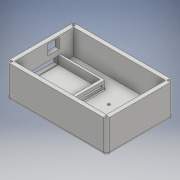
# Autodesk Inventor part: Back Plate test04
Saved by Autodesk Inventor 2018 (Build 220112000, 112)
## iProperties
Created: 2022-01-10
Part Number: Back Plate test04
Material: Generic
Document SubType Name: Modeling
Designer: Stewart Alexander
Density: 1 g/cm^3
Appearance: Default
Author: Stewart Alexander
Autodesk Inventor part; units mm, degrees
ref_plane "YZ Plane" through (0, 0, 0) normal (1, 0, 0) x (0, 1, 0)
ref_plane "XZ Plane" through (0, 0, 0) normal (0, 1, 0) x (-1, 0, 0)
ref_plane "XY Plane" through (0, 0, 0) normal (0, 0, 1) x (1, 0, 0)
sketch "Arduino Uno" plane through (0, 0, 0) normal (0, 0, 1) x (1, 0, 0)
  line L0 (0, 0) -> (68.6, 0)
  line L1 (68.6, 0) -> (68.6, 53.3)
  line L2 (68.6, 53.3) -> (0, 53.3)
  line L3 (0, 53.3) -> (0, 0)
  circle A0 centre (14, 2.5) radius 1.6
  circle A1 centre (15.3, 50.7) radius 1.6
  circle A2 centre (66.1, 5.1) radius 1.6
  circle A3 centre (66.1, 33) radius 1.6
  dimension "d6" = 68.6
  dimension "d7" = 53.3
  dimension "d8" = 3.2
  dimension "d12" = 14
  dimension "d13" = 2.5
  dimension "d14" = 3.2
  dimension "d15" = 1.3
  dimension "d16" = 3.2
  dimension "d18" = 2.5
  dimension "d19" = 5.1
  dimension "d20" = 3.2
  dimension "d21" = 27.9
  dimension "d22" = 2.5
  dimension "d26" = 2.6
  constraints: 8 end point, 4 centre point, 2 parallel, 1 horizontal, 1 perpendicular
  measures "d6" distance of L2.end L1.end
  measures "d7" distance of L0.end L1.end
  measures "d8" diameter of A0
  measures "d12" distance from line of L3 A0.centre
  measures "d13" distance from line of L0 A0.centre
  measures "d14" diameter of A1
  measures "d15" horizontal distance of A0.centre A1.centre
  measures "d16" diameter of A2
  measures "d18" distance from line of L1 A2.centre
  measures "d19" distance from line of L0 A2.centre
  measures "d20" diameter of A3
  measures "d21" distance of A2.centre A3.centre
  measures "d22" distance from line of L1 A3.centre
  measures "d26" distance from line of L2 A1.centre
sketch "Sketch2" plane through (0, 0, 0) normal (0, 0, 1) x (1, 0, 0)
  line L0 (-7.6136, -10.2044) -> (-7.6136, 63.0956)
  line L1 (-7.6136, 63.0956) -> (106.3864, 63.0956)
  line L2 (106.3864, 63.0956) -> (106.3864, -10.2044)
  line L3 (106.3864, -10.2044) -> (-7.6136, -10.2044)
  dimension "d29" = 114
  dimension "d39" = 73.3
  constraints: 8 end point, 3 perpendicular
  measures "d29" distance of L0.end L1.end
  measures "d39" distance of L0.start L0.end
extrude "Back Plate" add sketch "Sketch2" against normal blind 10
extrude "Uno Mounting Holes" cut sketch "Arduino Uno" against normal blind 5 contours A0 | A1 | A2 | A3
sketch "3.5\" TFT LCD Screen" plane through (0, 0, 0) normal (0, 0, 1) x (1, 0, 0)
  line L0 (88.6005, 0.0003) -> (88.6005, 53.3003)
  line L1 (88.6005, 53.3003) -> (10.6005, 53.3003)
  line L2 (10.6005, 53.3003) -> (10.6005, 0.0003)
  line L3 (10.6005, 0.0003) -> (88.6005, 0.0003)
  circle A0 centre (66.1, 5.1) radius 1.6 projected
  circle A1 centre (14, 2.5) radius 1.6 projected
  circle A2 centre (15.3, 50.7) radius 1.6 projected
  circle A3 centre (66.1, 33) radius 1.6 projected
  line L4 (-7.6136, -10.2044) -> (-7.6136, 63.0956) projected
  line L5 (106.3864, -10.2044) -> (-7.6136, -10.2044) projected
  line L6 (106.3864, 63.0956) -> (106.3864, -10.2044) projected
  line L7 (-7.6136, 63.0956) -> (106.3864, 63.0956) projected
  point P0 (0, 0)
  point P1 (68.6, 0)
  dimension "d35" = 78
  dimension "d36" = 53.3
  dimension "d37" = 78
  dimension "d38" = 53.3
  constraints: 8 end point
  measures "d35" distance of L2.end L0.start
  measures "d36" distance of L1.end L2.end
  measures "d37" distance of L0.end L1.end
  measures "d38" distance of L0.start L0.end
sketch "SD Card Slot" plane through (0, 0, 0) normal (0, 0, 1) x (1, 0, 0)
  line L0 (43.3864, 9.1) -> (-7.6136, 9.1)
  line L1 (-7.6136, 9.1) -> (-7.6136, 44.1)
  line L2 (-7.6136, 44.1) -> (43.3864, 44.1)
  line L3 (43.3864, 44.1) -> (43.3864, 9.1)
  circle A0 centre (14, 2.5) radius 1.6 projected
  line L4 (-7.6136, -10.2044) -> (-7.6136, 63.0956) projected
  circle A1 centre (15.3, 50.7) radius 1.6 projected
  point P0 (0, 0)
  dimension "d41" = 35
  dimension "d42" = 51
  dimension "d44" = 6.6
  dimension "d45" = 0
  constraints: 8 end point, 2 parallel, 1 horizontal, 1 perpendicular
  measures "d41" distance of L0.end L1.end
  measures "d42" distance of L0.start L0.end
  measures "d44" distance from line of L0 A0.centre
  measures "d45" distance between parallel lines of L4 L1
sketch "Sketch5" plane through (0, 0, 0) normal (0, 0, 1) x (1, 0, 0)
  line L0 (43.3864, 9.1) -> (-7.6136, 9.1) projected
  line L1 (43.3864, 44.1) -> (43.3864, 9.1) projected
  line L2 (-7.6136, 44.1) -> (43.3864, 44.1) projected
  line L3 (-7.6136, 9.1) -> (-7.6136, 44.1) projected
  line L4 (43.8864, 8.6) -> (43.8864, 44.6)
  line L5 (43.8864, 8.6) -> (-7.6136, 8.6)
  line L6 (-7.6136, -10.2044) -> (-7.6136, 63.0956) projected
  line L7 (43.8864, 44.6) -> (-7.6136, 44.6)
  line L8 (-7.6136, 44.6) -> (-7.6136, 47.1)
  line L9 (-7.6136, 47.1) -> (47.3864, 47.1)
  line L10 (-7.6136, 8.6) -> (-7.6136, 6.1)
  line L11 (-7.6136, 6.1) -> (47.3864, 6.1)
  line L12 (47.3864, 6.1) -> (47.3864, 47.1)
  point P0 (0, 0)
  dimension "d47" = 2.5
  dimension "d48" = 55
  dimension "d49" = 2.5
  dimension "d72" = 0.5
  dimension "d73" = 0.5
  dimension "d74" = 0.5
  constraints: 16 end point, 4 perpendicular, 3 point on line, 1 horizontal, 1 parallel
  measures "d47" distance of L7.end L8.end
  measures "d48" distance of L8.end L9.end
  measures "d49" distance of L5.end L10.end
  measures "d72" distance between parallel lines of L1 L4
  measures "d73" distance between parallel lines of L0 L5
  measures "d74" distance between parallel lines of L2 L7
extrude "SD Card Slot Slot" add sketch "Sketch5" along normal blind 10 contours L5 L4 L7 L6 L9 L12 L11
sketch "Sketch6" plane through (47.3864, 6.1, 0) normal (1, 0, 0) x (0, 0, -1)
  line L0 (0, 41) -> (0, 0) projected
  line L1 (0, 41) -> (-10, 41) projected
  line L2 (-10, 0) -> (-10, 41) projected
  line L3 (0, 0) -> (-10, 0) projected
  line L4 (-6, 37) -> (-4, 37)
  line L5 (-4, 37) -> (-4, 4)
  line L6 (-4, 4) -> (-6, 4)
  line L7 (-6, 4) -> (-6, 37)
  point P0 (0, -6.1)
  dimension "d52" = 4
  constraints: 8 end point, 3 other
  measures "d52" distance between parallel lines of L2 L7
extrude "SD Ribbon Slot" cut sketch "Sketch6" against normal through all contours L4 L5 L6 L7
fillet "1.2mm Fillet" radius 1.2 7 edges at (19.8864, 47.1, 0) (19.8864, 6.1, 0) (47.3864, 26.6, 0) (47.3864, 6.1, 5) (47.3864, 47.1, 5) (43.8864, 44.6, 5) (43.8864, 8.6, 5)
sketch "Sketch7" plane through (0, 0, 0) normal (0, 0, 1) x (1, 0, 0)
  line L0 (106.3864, -10.2044) -> (101.3864, -10.2044)
  line L1 (101.3864, -10.2044) -> (101.3864, -5.2044)
  line L2 (101.3864, -5.2044) -> (106.3864, -5.2044)
  line L3 (106.3864, -5.2044) -> (106.3864, -10.2044)
  line L4 (49.3864, -10.2044) -> (49.3864, 80.0118)
  line L5 (-7.6136, 63.0956) -> (106.3864, 63.0956) projected
  line L6 (106.3864, 26.4456) -> (-34.6963, 26.4456)
  line L7 (-7.6136, -10.2044) -> (-2.6136, -10.2044)
  line L8 (-2.6136, -10.2044) -> (-2.6136, -5.2044)
  line L9 (-2.6136, -5.2044) -> (-7.6136, -5.2044)
  line L10 (-7.6136, -5.2044) -> (-7.6136, -10.2044)
  line L11 (106.3864, 63.0956) -> (101.3864, 63.0956)
  line L12 (101.3864, 63.0956) -> (101.3864, 58.0956)
  line L13 (101.3864, 58.0956) -> (106.3864, 58.0956)
  line L14 (106.3864, 58.0956) -> (106.3864, 63.0956)
  line L15 (-7.6136, 63.0956) -> (-2.6136, 63.0956)
  line L16 (-2.6136, 63.0956) -> (-2.6136, 58.0956)
  line L17 (-2.6136, 58.0956) -> (-7.6136, 58.0956)
  line L18 (-7.6136, 58.0956) -> (-7.6136, 63.0956)
  point P0 (0, 0)
  point P1 (0, 52.8913)
  dimension "d56" = 5
  dimension "d57" = 5
  dimension "d58" = 57
  dimension "d59" = 36.65
  constraints: 36 end point, 11 symmetric about line, 2 parallel, 2 perpendicular, 1 horizontal
  measures "d56" distance of L1.end L2.end
  measures "d57" distance of L0.end L1.end
  measures "d58" distance of L0.start L4.start
  measures "d59" distance of L0.start L6.start
extrude "Pillars" [suppressed]
sketch "Sketch8" plane through (0, 0, 31) normal (0, 0, 1) x (1, 0, 0)
  line L0 (101.3864, -10.2044) -> (-2.6136, -10.2044) projected
  line L1 (-7.6136, -5.2044) -> (-2.6136, -5.2044) projected
  line L2 (101.3864, -10.2044) -> (-2.6136, -10.2044)
  line L3 (-2.6136, -10.2044) -> (-2.6136, -5.2044)
  line L4 (-2.6136, -5.2044) -> (101.3864, -5.2044)
  line L5 (101.3864, -5.2044) -> (101.3864, -10.2044)
  line L6 (101.3864, 63.0956) -> (101.3864, 58.0956) projected
  line L7 (106.3864, 63.0956) -> (106.3864, -10.2044) projected
  line L8 (101.3864, 58.0956) -> (106.3864, 58.0956)
  line L9 (106.3864, 58.0956) -> (106.3864, -5.2044)
  line L10 (106.3864, -5.2044) -> (101.3864, -5.2044)
  line L11 (101.3864, -5.2044) -> (101.3864, 58.0956)
  line L12 (-7.6136, 58.0956) -> (-2.6136, 58.0956) projected
  line L13 (-7.6136, 63.0956) -> (106.3864, 63.0956) projected
  line L14 (-2.6136, 58.0956) -> (101.3864, 58.0956)
  line L15 (101.3864, 58.0956) -> (101.3864, 63.0956)
  line L16 (101.3864, 63.0956) -> (-2.6136, 63.0956)
  line L17 (-2.6136, 63.0956) -> (-2.6136, 58.0956)
  line L18 (-2.6136, 58.0956) -> (-7.6136, 58.0956)
  line L19 (-7.6136, 58.0956) -> (-7.6136, -5.2044)
  line L20 (-7.6136, -5.2044) -> (-2.6136, -5.2044)
  line L21 (-2.6136, -5.2044) -> (-2.6136, 58.0956)
  point P0 (0, 0)
  constraints: 32 end point, 8 parallel, 4 horizontal, 4 perpendicular, 3 point on line
extrude "Beams (Will they print?)" [suppressed]
sketch "Sketch9" plane through (0, 0, 0) normal (0, 0, 1) x (1, 0, 0)
  line L0 (106.3864, 63.0956) -> (106.3864, -10.2044) projected
  line L1 (-7.6136, -10.2044) -> (-7.6136, 63.0956) projected
  line L2 (106.3864, -10.2044) -> (-7.6136, -10.2044)
  line L3 (-7.6136, -10.2044) -> (-7.6136, 63.0956)
  line L4 (-7.6136, 63.0956) -> (106.3864, 63.0956) projected
  line L5 (-7.6136, 63.0956) -> (106.3864, 63.0956)
  line L6 (106.3864, 63.0956) -> (106.3864, -10.2044)
  line L7 (106.3864, -10.2044) -> (106.3864, -15.2044)
  line L8 (106.3864, -15.2044) -> (-7.6136, -15.2044)
  line L9 (-7.6136, -15.2044) -> (-12.6136, -15.2044)
  line L10 (-12.6136, -15.2044) -> (-12.6136, 63.0956)
  line L11 (-12.6136, 63.0956) -> (-12.6136, 68.0956)
  line L12 (-12.6136, 68.0956) -> (106.3864, 68.0956)
  line L13 (106.3864, 68.0956) -> (111.3864, 68.0956)
  line L14 (111.3864, 68.0956) -> (111.3864, -15.2044)
  line L15 (111.3864, -15.2044) -> (106.3864, -15.2044)
  point P0 (0, 0)
  dimension "d64" = 5
  dimension "d65" = 5
  dimension "d66" = 5
  dimension "d67" = 5
  constraints: 26 end point, 8 point on line, 6 perpendicular, 2 collinear, 1 horizontal
  measures "d64" distance of L0.end L7.end
  measures "d65" distance of L8.end L9.end
  measures "d66" distance of L10.end L11.end
  measures "d67" distance of L12.end L13.end
extrude "Outer Walls (5mm Offset)" add sketch "Sketch9" along normal blind 31 and the other way blind 10
extrude "Extrusion9" [suppressed]
sketch "Sketch10" plane through (-12.6136, -15.2044, 31) normal (-1, 0, 0) x (0, 0, 1)
  line L0 (-31, 58.6044) -> (-21, 58.6044) projected
  line L1 (-29.8, 61.1044) -> (-29.8, 22.5044) projected
  line L2 (-21, 58.6044) -> (-21, 25.0044) projected
  line L3 (-21, 58.6044) -> (-21, 25.0044)
  line L4 (-21, 25.0044) -> (-29.8, 25.0044)
  line L5 (-29.8, 25.0044) -> (-29.8, 58.6044)
  line L6 (-29.8, 58.6044) -> (-21, 58.6044)
  line L7 (-31, 63.5044) -> (-31, 78.3) projected
  line L8 (-13.6, 59.5047) -> (-2.9, 59.5047)
  line L9 (-2.9, 59.5047) -> (-2.9, 47.5047)
  line L10 (-2.9, 47.5047) -> (-13.6, 47.5047)
  line L11 (-13.6, 47.5047) -> (-13.6, 59.5047)
  line L12 (-1.9, 46.5047) -> (-1.9, 60.5047)
  line L13 (-1.9, 60.5047) -> (-14.6, 60.5047)
  line L14 (-14.6, 60.5047) -> (-14.6, 46.5047)
  line L15 (-14.6, 46.5047) -> (-1.9, 46.5047)
  point P0 (-31, 15.2044)
  point P1 (-31, 68.5047)
  dimension "d82" = 10.7
  dimension "d83" = 12
  dimension "d84" = 1
  constraints: 24 end point, 7 perpendicular, 3 point on line, 2 collinear, 1 horizontal, 3 other
  measures "d82" distance of L8.start L8.end
  measures "d83" distance of L8.end L9.end
  measures "d84" distance between parallel lines of L9 L12
extrude "SD Card Opening" cut sketch "Sketch10" against normal blind 5 contours L0 L2 L4 L1 | L8 L9 L10 L11 | L15 L14 L13 L12
fillet "4mm Fillet" radius 4 8 edges at (-12.6136, 68.0956, 10.5) (-12.6136, -15.2044, 10.5) (111.3864, -15.2044, 10.5) (111.3864, 68.0956, 10.5) (49.3864, 68.0956, -10) (-12.6136, 26.4456, -10) (49.3864, -15.2044, -10) (111.3864, 26.4456, -10)
sketch "Sketch11" plane through (0, 0, 0) normal (0, 0, 1) x (1, 0, 0)
  line L0 (98.4778, 47.4456) -> (98.4778, 5.4456) construction
  line L1 (98.4778, 5.4456) -> (86.054, 5.4456) construction
  line L2 (86.054, 5.4456) -> (86.054, 47.4456) construction
  line L3 (86.054, 47.4456) -> (98.4778, 47.4456) construction
  line L4 (-8.6136, 68.0956) -> (107.3864, 68.0956) projected
  line L5 (107.3864, 68.0956) -> (107.3864, 26.4456)
  line L6 (107.3864, 26.4456) -> (48.9636, 26.4456)
  line L7 (94.9648, 45.4666) -> (98.011, 44.7345)
  line L8 (98.011, 44.7345) -> (98.011, 45.124)
  line L9 (98.011, 45.124) -> (98.4778, 45.0166)
  line L10 (98.4778, 45.0166) -> (98.4778, 42.1518)
  line L11 (98.4778, 42.1518) -> (97.2789, 42.454)
  line L12 (97.2789, 42.454) -> (97.2789, 42.9276)
  line L13 (97.2789, 42.9276) -> (98.011, 42.7429)
  line L14 (98.011, 42.7429) -> (98.011, 44.1534)
  line L15 (98.011, 44.1534) -> (96.7952, 44.4456)
  line L16 (96.7952, 44.4456) -> (96.7952, 43.25)
  line L17 (96.7952, 43.25) -> (96.3284, 43.3575)
  line L18 (96.3284, 43.3575) -> (96.3284, 44.5565)
  line L19 (96.3284, 44.5565) -> (94.9648, 44.8856)
  line L20 (94.9648, 44.8856) -> (94.9648, 44.4591)
  line L21 (94.9648, 44.4591) -> (94.498, 44.5665)
  line L22 (94.498, 44.5665) -> (94.498, 45.9301)
  line L23 (94.498, 45.9301) -> (94.9648, 45.8226)
  line L24 (94.9648, 45.8226) -> (94.9648, 45.4666)
  spline S0 degree 2 poles (95.613, 42.5313) (96.0396, 42.5313) (96.8255, 42.1316) (97.3427, 41.3323) (97.3427, 40.8352) knots 0 0 0 1 2 3 3 3
  spline S1 degree 2 poles (97.3427, 40.8352) (97.3427, 40.2575) (96.6676, 39.6362) (96.1538, 39.6362) knots 0 0 0 1 2 2 2
  spline S2 degree 2 poles (96.1538, 39.6362) (95.7474, 39.6362) (94.8943, 40.0325) (94.4174, 40.8554) (94.4174, 41.3155) knots 0 0 0 1 2 3 3 3
  spline S3 degree 2 poles (94.4174, 41.3155) (94.4174, 41.8495) (95.0488, 42.5313) (95.613, 42.5313) knots 0 0 0 1 2 2 2
  spline S4 degree 2 poles (95.6634, 41.9536) (94.9145, 41.9536) (94.9145, 41.2617) knots 0 0 0 1 1 1
  spline S5 degree 2 poles (94.9145, 41.2617) (94.9145, 40.7748) (95.66, 40.187) (96.1504, 40.187) knots 0 0 0 1 2 2 2
  spline S6 degree 2 poles (96.1504, 40.187) (96.4661, 40.187) (96.8456, 40.59) (96.8456, 40.9192) knots 0 0 0 1 2 2 2
  spline S7 degree 2 poles (96.8456, 40.9192) (96.8456, 41.3894) (96.1235, 41.9536) (95.6634, 41.9536) knots 0 0 0 1 2 2 2
  line L25 (94.9648, 38.5581) -> (94.9648, 38.1014)
  line L26 (94.9648, 38.1014) -> (94.498, 38.2122)
  line L27 (94.498, 38.2122) -> (94.498, 39.5489)
  line L28 (94.498, 39.5489) -> (94.9648, 39.4414)
  line L29 (94.9648, 39.4414) -> (94.9648, 39.0787)
  line L30 (94.9648, 39.0787) -> (96.7986, 38.6656)
  line L31 (96.7986, 38.6656) -> (96.7986, 39.0955)
  line L32 (96.7986, 39.0955) -> (97.2654, 38.9813)
  line L33 (97.2654, 38.9813) -> (97.2654, 38.0846)
  line L34 (97.2654, 38.0846) -> (96.4829, 38.2626)
  spline S8 degree 2 poles (96.4829, 38.2626) (96.9161, 38.0006) (97.3091, 37.4028) (97.3091, 36.9998) knots 0 0 0 1 2 2 2
  line L35 (97.3091, 36.9998) -> (97.3091, 36.8755)
  line L36 (97.3091, 36.8755) -> (96.7986, 36.9964)
  spline S9 degree 2 poles (96.7986, 36.9964) (96.8087, 37.0737) (96.8087, 37.1274) knots 0 0 0 1 1 1
  spline S10 degree 2 poles (96.8087, 37.1274) (96.8087, 37.4935) (96.4728, 38.0275) (95.9019, 38.3465) (95.4619, 38.4473) knots 0 0 0 1 2 3 3 3
  line L37 (95.4619, 38.4473) -> (94.9648, 38.5581)
  line L38 (94.9648, 33.2315) -> (94.9648, 32.8856)
  line L39 (94.9648, 32.8856) -> (94.498, 32.983)
  line L40 (94.498, 32.983) -> (94.498, 33.8293)
  line L41 (94.498, 33.8293) -> (94.8842, 33.742)
  spline S11 degree 2 poles (94.8842, 33.742) (94.451, 34.1383) (94.451, 34.6354) knots 0 0 0 1 1 1
  spline S12 degree 2 poles (94.451, 34.6354) (94.451, 34.9578) (94.8909, 35.4683) (95.2604, 35.4683) knots 0 0 0 1 2 2 2
  spline S13 degree 2 poles (95.2604, 35.4683) (95.6768, 35.4683) (96.2243, 34.7932) (96.2243, 34.2962) knots 0 0 0 1 2 2 2
  spline S14 degree 2 poles (96.2243, 34.2962) (96.2243, 33.9099) (96.0228, 33.5271) knots 0 0 0 1 1 1
  line L42 (96.0228, 33.5271) -> (96.3284, 33.4532)
  spline S15 degree 2 poles (96.3284, 33.4532) (96.4896, 33.4162) (96.5568, 33.4162) knots 0 0 0 1 1 1
  spline S16 degree 2 poles (96.5568, 33.4162) (96.7381, 33.4162) (96.9296, 33.7017) (96.9296, 33.9099) knots 0 0 0 1 2 2 2
  spline S17 degree 2 poles (96.9296, 33.9099) (96.9296, 34.313) (96.5366, 34.5884) knots 0 0 0 1 1 1
  line L43 (96.5366, 34.5884) -> (96.7348, 35.0216)
  spline S18 degree 2 poles (96.7348, 35.0216) (96.9934, 34.8537) (97.3427, 34.2021) (97.3427, 33.8159) knots 0 0 0 1 2 2 2
  spline S19 degree 2 poles (97.3427, 33.8159) (97.3427, 33.3793) (96.9665, 32.899) (96.6642, 32.899) knots 0 0 0 1 2 2 2
  spline S20 degree 2 poles (96.6642, 32.899) (96.4795, 32.899) (96.1941, 32.9628) knots 0 0 0 1 1 1
  line L44 (96.1941, 32.9628) -> (94.9648, 33.2315)
  line L45 (95.6433, 33.6077) -> (95.7004, 33.7319)
  spline S21 degree 2 poles (95.7004, 33.7319) (95.828, 34.0174) (95.828, 34.2559) knots 0 0 0 1 1 1
  spline S22 degree 2 poles (95.828, 34.2559) (95.828, 34.5716) (95.5022, 34.9544) (95.2772, 34.9544) knots 0 0 0 1 2 2 2
  spline S23 degree 2 poles (95.2772, 34.9544) (95.0857, 34.9544) (94.8641, 34.6891) (94.8641, 34.4708) knots 0 0 0 1 2 2 2
  spline S24 degree 2 poles (94.8641, 34.4708) (94.8641, 34.135) (95.2268, 33.7118) knots 0 0 0 1 1 1
  line L46 (95.2268, 33.7118) -> (95.6433, 33.6077)
  line L47 (94.9648, 32.1635) -> (98.011, 31.4314)
  line L48 (98.011, 31.4314) -> (98.011, 31.8041)
  line L49 (98.011, 31.8041) -> (98.4778, 31.6967)
  line L50 (98.4778, 31.6967) -> (98.4778, 30.7999)
  line L51 (98.4778, 30.7999) -> (94.9648, 31.6463)
  line L52 (94.9648, 31.6463) -> (94.9648, 31.2701)
  line L53 (94.9648, 31.2701) -> (94.498, 31.381)
  line L54 (94.498, 31.381) -> (94.498, 32.59)
  line L55 (94.498, 32.59) -> (94.9648, 32.4826)
  line L56 (94.9648, 32.4826) -> (94.9648, 32.1635)
  line L57 (94.9648, 30.5178) -> (98.011, 29.7857)
  line L58 (98.011, 29.7857) -> (98.011, 30.1585)
  line L59 (98.011, 30.1585) -> (98.4778, 30.051)
  line L60 (98.4778, 30.051) -> (98.4778, 29.1543)
  line L61 (98.4778, 29.1543) -> (94.9648, 30.0006)
  line L62 (94.9648, 30.0006) -> (94.9648, 29.6245)
  line L63 (94.9648, 29.6245) -> (94.498, 29.7353)
  line L64 (94.498, 29.7353) -> (94.498, 30.9444)
  line L65 (94.498, 30.9444) -> (94.9648, 30.8369)
  line L66 (94.9648, 30.8369) -> (94.9648, 30.5178)
  line L67 (97.2654, 26.4204) -> (97.2654, 26.0208)
  line L68 (97.2654, 26.0208) -> (96.7986, 26.1282)
  line L69 (96.7986, 26.1282) -> (96.7986, 26.5313)
  line L70 (96.7986, 26.5313) -> (95.4955, 26.847)
  spline S25 degree 2 poles (95.4955, 26.847) (95.1428, 26.9343) (95.0555, 26.9343) knots 0 0 0 1 1 1
  spline S26 degree 2 poles (95.0555, 26.9343) (94.8607, 26.9343) (94.8607, 26.7261) knots 0 0 0 1 1 1
  spline S27 degree 2 poles (94.8607, 26.7261) (94.8607, 26.585) (95.0219, 26.2962) knots 0 0 0 1 1 1
  line L71 (95.0219, 26.2962) -> (94.545, 26.407)
  spline S28 degree 2 poles (94.545, 26.407) (94.4174, 26.669) (94.4174, 26.9175) knots 0 0 0 1 1 1
  spline S29 degree 2 poles (94.4174, 26.9175) (94.4174, 27.1526) (94.7197, 27.4448) (94.9951, 27.4448) knots 0 0 0 1 2 2 2
  spline S30 degree 2 poles (94.9951, 27.4448) (95.1831, 27.4448) (95.8179, 27.2869) knots 0 0 0 1 1 1
  line L72 (95.8179, 27.2869) -> (96.7986, 27.0518)
  line L73 (96.7986, 27.0518) -> (96.7986, 27.3575)
  line L74 (96.7986, 27.3575) -> (97.2654, 27.25)
  line L75 (97.2654, 27.25) -> (97.2654, 26.9376)
  line L76 (97.2654, 26.9376) -> (97.8162, 26.8033)
  line L77 (97.8162, 26.8033) -> (98.3099, 26.1652)
  line L78 (98.3099, 26.1652) -> (97.2654, 26.4204)
  line L79 (94.9648, 23.5691) -> (94.9648, 23.156)
  line L80 (94.9648, 23.156) -> (94.498, 23.2668)
  line L81 (94.498, 23.2668) -> (94.498, 24.2005)
  line L82 (94.498, 24.2005) -> (96.0328, 23.8377)
  spline S31 degree 2 poles (96.0328, 23.8377) (96.4459, 23.7437) (96.5333, 23.7437) knots 0 0 0 1 1 1
  spline S32 degree 2 poles (96.5333, 23.7437) (96.8187, 23.7437) (96.8187, 24.0392) knots 0 0 0 1 1 1
  spline S33 degree 2 poles (96.8187, 24.0392) (96.8187, 24.3146) (96.4459, 24.8621) knots 0 0 0 1 1 1
  line L83 (96.4459, 24.8621) -> (94.9648, 25.2214)
  line L84 (94.9648, 25.2214) -> (94.9648, 24.8083)
  line L85 (94.9648, 24.8083) -> (94.498, 24.9158)
  line L86 (94.498, 24.9158) -> (94.498, 26.1786)
  line L87 (94.498, 26.1786) -> (94.9648, 26.0712)
  line L88 (94.9648, 26.0712) -> (94.9648, 25.7387)
  line L89 (94.9648, 25.7387) -> (98.011, 25.0065)
  line L90 (98.011, 25.0065) -> (98.011, 25.3726)
  line L91 (98.011, 25.3726) -> (98.4778, 25.2651)
  line L92 (98.4778, 25.2651) -> (98.4778, 24.3751)
  line L93 (98.4778, 24.3751) -> (96.9396, 24.7445)
  spline S34 degree 2 poles (96.9396, 24.7445) (97.3091, 24.224) (97.3091, 23.8478) knots 0 0 0 1 1 1
  spline S35 degree 2 poles (97.3091, 23.8478) (97.3091, 23.5388) (96.9161, 23.213) (96.6676, 23.213) knots 0 0 0 1 2 2 2
  spline S36 degree 2 poles (96.6676, 23.213) (96.4829, 23.213) (95.9858, 23.3306) knots 0 0 0 1 1 1
  line L94 (95.9858, 23.3306) -> (94.9648, 23.5691)
  line L95 (95.7541, 19.8579) -> (95.7541, 22.0308)
  spline S37 degree 2 poles (95.7541, 22.0308) (95.6701, 22.051) (95.5962, 22.051) knots 0 0 0 1 1 1
  spline S38 degree 2 poles (95.5962, 22.051) (95.2537, 22.051) (94.8708, 21.6581) (94.8708, 21.3591) knots 0 0 0 1 2 2 2
  spline S39 degree 2 poles (94.8708, 21.3591) (94.8708, 20.946) (95.2637, 20.6572) knots 0 0 0 1 1 1
  line L96 (95.2637, 20.6572) -> (95.032, 20.1165)
  spline S40 degree 2 poles (95.032, 20.1165) (94.7633, 20.2811) (94.4174, 20.9662) (94.4174, 21.3558) knots 0 0 0 1 2 2 2
  spline S41 degree 2 poles (94.4174, 21.3558) (94.4174, 21.9536) (95.1093, 22.6152) (95.65, 22.6152) knots 0 0 0 1 2 2 2
  spline S42 degree 2 poles (95.65, 22.6152) (96.0832, 22.6152) (96.8523, 22.1786) (97.3427, 21.4465) (97.3427, 21.0099) knots 0 0 0 1 2 3 3 3
  spline S43 degree 2 poles (97.3427, 21.0099) (97.3427, 20.4826) (96.6542, 19.8176) (96.0967, 19.8176) knots 0 0 0 1 2 2 2
  spline S44 degree 2 poles (96.0967, 19.8176) (95.9187, 19.8176) (95.7541, 19.8579) knots 0 0 0 1 1 1
  spline S45 degree 2 poles (96.1437, 20.3482) (96.231, 20.3382) (96.2881, 20.3382) knots 0 0 0 1 1 1
  spline S46 degree 2 poles (96.2881, 20.3382) (96.5165, 20.3382) (96.8893, 20.7009) (96.8893, 21.0031) knots 0 0 0 1 2 2 2
  spline S47 degree 2 poles (96.8893, 21.0031) (96.8893, 21.3088) (96.4862, 21.8025) (96.1437, 21.9267) knots 0 0 0 1 2 2 2
  line L97 (96.1437, 21.9267) -> (96.1437, 20.3482)
  line L98 (94.9648, 17.8025) -> (98.011, 17.0703)
  line L99 (98.011, 17.0703) -> (98.011, 17.4599)
  line L100 (98.011, 17.4599) -> (98.4778, 17.3491)
  line L101 (98.4778, 17.3491) -> (98.4778, 16.4423)
  line L102 (98.4778, 16.4423) -> (96.9329, 16.8117)
  spline S48 degree 2 poles (96.9329, 16.8117) (97.3427, 16.402) (97.3427, 15.868) knots 0 0 0 1 1 1
  spline S49 degree 2 poles (97.3427, 15.868) (97.3427, 15.391) (96.6978, 14.7664) (96.1571, 14.7664) knots 0 0 0 1 2 2 2
  spline S50 degree 2 poles (96.1571, 14.7664) (95.4417, 14.7664) (94.451, 15.6429) (94.451, 16.3079) knots 0 0 0 1 2 2 2
  spline S51 degree 2 poles (94.451, 16.3079) (94.451, 16.9125) (94.9648, 17.2853) knots 0 0 0 1 1 1
  line L103 (94.9648, 17.2853) -> (94.498, 17.3961)
  line L104 (94.498, 17.3961) -> (94.498, 18.2256)
  line L105 (94.498, 18.2256) -> (94.9648, 18.1182)
  line L106 (94.9648, 18.1182) -> (94.9648, 17.8025)
  spline S52 degree 2 poles (95.65, 17.0871) (95.3007, 17.0871) (94.9044, 16.6908) (94.9044, 16.3785) knots 0 0 0 1 2 2 2
  spline S53 degree 2 poles (94.9044, 16.3785) (94.9044, 15.915) (95.6466, 15.2903) (96.1269, 15.2903) knots 0 0 0 1 2 2 2
  spline S54 degree 2 poles (96.1269, 15.2903) (96.4862, 15.2903) (96.8725, 15.6967) (96.8725, 16.009) knots 0 0 0 1 2 2 2
  spline S55 degree 2 poles (96.8725, 16.009) (96.8725, 16.4759) (96.0899, 17.0871) (95.65, 17.0871) knots 0 0 0 1 2 2 2
  line L107 (95.7541, 11.559) -> (95.7541, 13.7319)
  spline S56 degree 2 poles (95.7541, 13.7319) (95.6701, 13.7521) (95.5962, 13.7521) knots 0 0 0 1 1 1
  spline S57 degree 2 poles (95.5962, 13.7521) (95.2537, 13.7521) (94.8708, 13.3591) (94.8708, 13.0602) knots 0 0 0 1 2 2 2
  spline S58 degree 2 poles (94.8708, 13.0602) (94.8708, 12.6471) (95.2637, 12.3583) knots 0 0 0 1 1 1
  line L108 (95.2637, 12.3583) -> (95.032, 11.8176)
  spline S59 degree 2 poles (95.032, 11.8176) (94.7633, 11.9821) (94.4174, 12.6673) (94.4174, 13.0569) knots 0 0 0 1 2 2 2
  spline S60 degree 2 poles (94.4174, 13.0569) (94.4174, 13.6547) (95.1093, 14.3163) (95.65, 14.3163) knots 0 0 0 1 2 2 2
  spline S61 degree 2 poles (95.65, 14.3163) (96.0832, 14.3163) (96.8523, 13.8797) (97.3427, 13.1476) (97.3427, 12.7109) knots 0 0 0 1 2 3 3 3
  spline S62 degree 2 poles (97.3427, 12.7109) (97.3427, 12.1837) (96.6542, 11.5187) (96.0967, 11.5187) knots 0 0 0 1 2 2 2
  spline S63 degree 2 poles (96.0967, 11.5187) (95.9187, 11.5187) (95.7541, 11.559) knots 0 0 0 1 1 1
  spline S64 degree 2 poles (96.1437, 12.0493) (96.231, 12.0392) (96.2881, 12.0392) knots 0 0 0 1 1 1
  spline S65 degree 2 poles (96.2881, 12.0392) (96.5165, 12.0392) (96.8893, 12.402) (96.8893, 12.7042) knots 0 0 0 1 2 2 2
  spline S66 degree 2 poles (96.8893, 12.7042) (96.8893, 13.0099) (96.4862, 13.5036) (96.1437, 13.6278) knots 0 0 0 1 2 2 2
  line L109 (96.1437, 13.6278) -> (96.1437, 12.0493)
  line L110 (95.2705, 11.2534) -> (95.2705, 10.7832)
  spline S67 degree 2 poles (95.2705, 10.7832) (95.0757, 10.7832) (94.8641, 10.4406) (94.8641, 10.1652) knots 0 0 0 1 2 2 2
  spline S68 degree 2 poles (94.8641, 10.1652) (94.8641, 9.9099) (95.0689, 9.6345) (95.2201, 9.6345) knots 0 0 0 1 2 2 2
  spline S69 degree 2 poles (95.2201, 9.6345) (95.3578, 9.6345) (95.566, 9.8764) (95.6836, 10.1786) knots 0 0 0 1 2 2 2
  spline S70 degree 2 poles (95.6836, 10.1786) (95.8011, 10.4842) (95.9892, 10.7999) (96.3217, 11.0048) (96.5098, 11.0048) knots 0 0 0 1 2 3 3 3
  spline S71 degree 2 poles (96.5098, 11.0048) (96.8288, 11.0048) (97.3091, 10.4742) (97.3091, 10.0073) knots 0 0 0 1 2 2 2
  spline S72 degree 2 poles (97.3091, 10.0073) (97.3091, 9.5741) (97.0673, 9.292) knots 0 0 0 1 1 1
  line L111 (97.0673, 9.292) -> (97.2654, 9.2349)
  line L112 (97.2654, 9.2349) -> (97.2654, 8.7748)
  line L113 (97.2654, 8.7748) -> (96.4963, 8.9561)
  line L114 (96.4963, 8.9561) -> (96.4963, 9.4196)
  spline S73 degree 2 poles (96.4963, 9.4196) (96.7079, 9.4263) (96.8859, 9.7958) (96.8859, 10.0174) knots 0 0 0 1 2 2 2
  spline S74 degree 2 poles (96.8859, 10.0174) (96.8859, 10.2458) (96.7045, 10.5044) (96.5669, 10.5044) knots 0 0 0 1 2 2 2
  spline S75 degree 2 poles (96.5669, 10.5044) (96.4527, 10.5044) (96.3082, 10.3499) (96.2243, 10.1316) knots 0 0 0 1 2 2 2
  spline S76 degree 2 poles (96.2243, 10.1316) (95.9892, 9.5136) (95.5593, 9.1207) (95.257, 9.1207) knots 0 0 0 1 2 2 2
  spline S77 degree 2 poles (95.257, 9.1207) (94.8943, 9.1207) (94.451, 9.6782) (94.451, 10.2156) knots 0 0 0 1 2 2 2
  spline S78 degree 2 poles (94.451, 10.2156) (94.451, 10.7193) (94.6794, 10.9276) knots 0 0 0 1 1 1
  line L115 (94.6794, 10.9276) -> (94.498, 10.9679)
  line L116 (94.498, 10.9679) -> (94.498, 11.4381)
  line L117 (94.498, 11.4381) -> (95.2705, 11.2534)
  line L118 (97.2654, 7.4515) -> (97.2654, 7.0518)
  line L119 (97.2654, 7.0518) -> (96.7986, 7.1593)
  line L120 (96.7986, 7.1593) -> (96.7986, 7.5623)
  line L121 (96.7986, 7.5623) -> (95.4955, 7.878)
  spline S79 degree 2 poles (95.4955, 7.878) (95.1428, 7.9654) (95.0555, 7.9654) knots 0 0 0 1 1 1
  spline S80 degree 2 poles (95.0555, 7.9654) (94.8607, 7.9654) (94.8607, 7.7571) knots 0 0 0 1 1 1
  spline S81 degree 2 poles (94.8607, 7.7571) (94.8607, 7.6161) (95.0219, 7.3272) knots 0 0 0 1 1 1
  line L122 (95.0219, 7.3272) -> (94.545, 7.4381)
  spline S82 degree 2 poles (94.545, 7.4381) (94.4174, 7.7) (94.4174, 7.9486) knots 0 0 0 1 1 1
  spline S83 degree 2 poles (94.4174, 7.9486) (94.4174, 8.1837) (94.7197, 8.4759) (94.9951, 8.4759) knots 0 0 0 1 2 2 2
  spline S84 degree 2 poles (94.9951, 8.4759) (95.1831, 8.4759) (95.8179, 8.318) knots 0 0 0 1 1 1
  line L123 (95.8179, 8.318) -> (96.7986, 8.0829)
  line L124 (96.7986, 8.0829) -> (96.7986, 8.3885)
  line L125 (96.7986, 8.3885) -> (97.2654, 8.2811)
  line L126 (97.2654, 8.2811) -> (97.2654, 7.9687)
  line L127 (97.2654, 7.9687) -> (97.8162, 7.8344)
  line L128 (97.8162, 7.8344) -> (98.3099, 7.1963)
  line L129 (98.3099, 7.1963) -> (97.2654, 7.4515)
  line L130 (90.6843, 39.0334) -> (90.6843, 38.1635)
  line L131 (90.6843, 38.1635) -> (90.3451, 38.2408)
  spline S85 degree 2 poles (90.3451, 38.2408) (90.728, 37.69) (90.728, 37.2735) knots 0 0 0 1 1 1
  spline S86 degree 2 poles (90.728, 37.2735) (90.728, 37.0518) (90.4694, 36.7193) (90.2679, 36.6589) knots 0 0 0 1 2 2 2
  spline S87 degree 2 poles (90.2679, 36.6589) (90.728, 36.0812) (90.728, 35.6345) knots 0 0 0 1 1 1
  spline S88 degree 2 poles (90.728, 35.6345) (90.728, 35.3121) (90.3249, 34.9863) (90.0898, 34.9863) knots 0 0 0 1 2 2 2
  spline S89 degree 2 poles (90.0898, 34.9863) (89.9085, 34.9863) (89.5223, 35.077) knots 0 0 0 1 1 1
  line L132 (89.5223, 35.077) -> (88.3837, 35.3491)
  line L133 (88.3837, 35.3491) -> (88.3837, 34.9393)
  line L134 (88.3837, 34.9393) -> (87.9169, 35.0468)
  line L135 (87.9169, 35.0468) -> (87.9169, 35.9771)
  line L136 (87.9169, 35.9771) -> (89.5827, 35.5808)
  spline S90 degree 2 poles (89.5827, 35.5808) (89.8346, 35.5204) (89.9454, 35.5204) knots 0 0 0 1 1 1
  spline S91 degree 2 poles (89.9454, 35.5204) (90.2376, 35.5204) (90.2376, 35.8092) knots 0 0 0 1 1 1
  spline S92 degree 2 poles (90.2376, 35.8092) (90.2376, 36.1148) (89.8615, 36.6589) knots 0 0 0 1 1 1
  line L137 (89.8615, 36.6589) -> (88.3837, 37.0048)
  line L138 (88.3837, 37.0048) -> (88.3837, 36.5884)
  line L139 (88.3837, 36.5884) -> (87.9169, 36.6992)
  line L140 (87.9169, 36.6992) -> (87.9169, 37.6329)
  line L141 (87.9169, 37.6329) -> (89.6163, 37.2366)
  spline S93 degree 2 poles (89.6163, 37.2366) (89.8648, 37.1761) (89.9454, 37.1761) knots 0 0 0 1 1 1
  spline S94 degree 2 poles (89.9454, 37.1761) (90.0731, 37.1761) (90.2376, 37.3507) (90.2376, 37.4683) knots 0 0 0 1 2 2 2
  spline S95 degree 2 poles (90.2376, 37.4683) (90.2376, 37.7773) (89.8581, 38.3516) knots 0 0 0 1 1 1
  line L142 (89.8581, 38.3516) -> (88.3837, 38.6807)
  line L143 (88.3837, 38.6807) -> (88.3837, 38.2676)
  line L144 (88.3837, 38.2676) -> (87.9169, 38.3818)
  line L145 (87.9169, 38.3818) -> (87.9169, 39.6278)
  line L146 (87.9169, 39.6278) -> (88.3837, 39.5204)
  line L147 (88.3837, 39.5204) -> (88.3837, 39.1979)
  line L148 (88.3837, 39.1979) -> (90.2175, 38.7848)
  line L149 (90.2175, 38.7848) -> (90.2175, 39.1408)
  line L150 (90.2175, 39.1408) -> (90.6843, 39.0334)
  line L151 (89.173, 31.6547) -> (89.173, 33.8277)
  spline S96 degree 2 poles (89.173, 33.8277) (89.089, 33.8478) (89.0151, 33.8478) knots 0 0 0 1 1 1
  spline S97 degree 2 poles (89.0151, 33.8478) (88.6726, 33.8478) (88.2897, 33.4549) (88.2897, 33.156) knots 0 0 0 1 2 2 2
  spline S98 degree 2 poles (88.2897, 33.156) (88.2897, 32.7429) (88.6826, 32.454) knots 0 0 0 1 1 1
  line L152 (88.6826, 32.454) -> (88.4509, 31.9133)
  spline S99 degree 2 poles (88.4509, 31.9133) (88.1822, 32.0779) (87.8363, 32.763) (87.8363, 33.1526) knots 0 0 0 1 2 2 2
  spline S100 degree 2 poles (87.8363, 33.1526) (87.8363, 33.7504) (88.5281, 34.412) (89.0689, 34.412) knots 0 0 0 1 2 2 2
  spline S101 degree 2 poles (89.0689, 34.412) (89.5021, 34.412) (90.2712, 33.9754) (90.7616, 33.2433) (90.7616, 32.8067) knots 0 0 0 1 2 3 3 3
  spline S102 degree 2 poles (90.7616, 32.8067) (90.7616, 32.2794) (90.0731, 31.6144) (89.5155, 31.6144) knots 0 0 0 1 2 2 2
  spline S103 degree 2 poles (89.5155, 31.6144) (89.3375, 31.6144) (89.173, 31.6547) knots 0 0 0 1 1 1
  spline S104 degree 2 poles (89.5626, 32.145) (89.6499, 32.135) (89.707, 32.135) knots 0 0 0 1 1 1
  spline S105 degree 2 poles (89.707, 32.135) (89.9354, 32.135) (90.3082, 32.4977) (90.3082, 32.7999) knots 0 0 0 1 2 2 2
  spline S106 degree 2 poles (90.3082, 32.7999) (90.3082, 33.1056) (89.9051, 33.5993) (89.5626, 33.7235) knots 0 0 0 1 2 2 2
  line L153 (89.5626, 33.7235) -> (89.5626, 32.145)
  line L154 (90.6843, 30.8587) -> (90.6843, 29.9889)
  line L155 (90.6843, 29.9889) -> (90.3451, 30.0661)
  spline S107 degree 2 poles (90.3451, 30.0661) (90.728, 29.5153) (90.728, 29.0989) knots 0 0 0 1 1 1
  spline S108 degree 2 poles (90.728, 29.0989) (90.728, 28.8772) (90.4694, 28.5447) (90.2679, 28.4842) knots 0 0 0 1 2 2 2
  spline S109 degree 2 poles (90.2679, 28.4842) (90.728, 27.9066) (90.728, 27.4599) knots 0 0 0 1 1 1
  spline S110 degree 2 poles (90.728, 27.4599) (90.728, 27.1375) (90.3249, 26.8117) (90.0898, 26.8117) knots 0 0 0 1 2 2 2
  spline S111 degree 2 poles (90.0898, 26.8117) (89.9085, 26.8117) (89.5223, 26.9024) knots 0 0 0 1 1 1
  line L156 (89.5223, 26.9024) -> (88.3837, 27.1744)
  line L157 (88.3837, 27.1744) -> (88.3837, 26.7647)
  line L158 (88.3837, 26.7647) -> (87.9169, 26.8722)
  line L159 (87.9169, 26.8722) -> (87.9169, 27.8025)
  line L160 (87.9169, 27.8025) -> (89.5827, 27.4062)
  spline S112 degree 2 poles (89.5827, 27.4062) (89.8346, 27.3457) (89.9454, 27.3457) knots 0 0 0 1 1 1
  spline S113 degree 2 poles (89.9454, 27.3457) (90.2376, 27.3457) (90.2376, 27.6345) knots 0 0 0 1 1 1
  spline S114 degree 2 poles (90.2376, 27.6345) (90.2376, 27.9402) (89.8615, 28.4842) knots 0 0 0 1 1 1
  line L161 (89.8615, 28.4842) -> (88.3837, 28.8302)
  line L162 (88.3837, 28.8302) -> (88.3837, 28.4137)
  line L163 (88.3837, 28.4137) -> (87.9169, 28.5246)
  line L164 (87.9169, 28.5246) -> (87.9169, 29.4582)
  line L165 (87.9169, 29.4582) -> (89.6163, 29.0619)
  spline S115 degree 2 poles (89.6163, 29.0619) (89.8648, 29.0015) (89.9454, 29.0015) knots 0 0 0 1 1 1
  spline S116 degree 2 poles (89.9454, 29.0015) (90.0731, 29.0015) (90.2376, 29.1761) (90.2376, 29.2937) knots 0 0 0 1 2 2 2
  spline S117 degree 2 poles (90.2376, 29.2937) (90.2376, 29.6026) (89.8581, 30.1769) knots 0 0 0 1 1 1
  line L166 (89.8581, 30.1769) -> (88.3837, 30.5061)
  line L167 (88.3837, 30.5061) -> (88.3837, 30.093)
  line L168 (88.3837, 30.093) -> (87.9169, 30.2072)
  line L169 (87.9169, 30.2072) -> (87.9169, 31.4532)
  line L170 (87.9169, 31.4532) -> (88.3837, 31.3457)
  line L171 (88.3837, 31.3457) -> (88.3837, 31.0233)
  line L172 (88.3837, 31.0233) -> (90.2175, 30.6102)
  line L173 (90.2175, 30.6102) -> (90.2175, 30.9662)
  line L174 (90.2175, 30.9662) -> (90.6843, 30.8587)
  spline S118 degree 2 poles (89.0319, 26.2643) (89.4584, 26.2643) (90.2443, 25.8646) (90.7616, 25.0653) (90.7616, 24.5682) knots 0 0 0 1 2 3 3 3
  spline S119 degree 2 poles (90.7616, 24.5682) (90.7616, 23.9905) (90.0865, 23.3692) (89.5726, 23.3692) knots 0 0 0 1 2 2 2
  spline S120 degree 2 poles (89.5726, 23.3692) (89.1663, 23.3692) (88.3132, 23.7655) (87.8363, 24.5884) (87.8363, 25.0485) knots 0 0 0 1 2 3 3 3
  spline S121 degree 2 poles (87.8363, 25.0485) (87.8363, 25.5825) (88.4677, 26.2643) (89.0319, 26.2643) knots 0 0 0 1 2 2 2
  spline S122 degree 2 poles (89.0823, 25.6866) (88.3333, 25.6866) (88.3333, 24.9947) knots 0 0 0 1 1 1
  spline S123 degree 2 poles (88.3333, 24.9947) (88.3333, 24.5078) (89.0789, 23.92) (89.5693, 23.92) knots 0 0 0 1 2 2 2
  spline S124 degree 2 poles (89.5693, 23.92) (89.885, 23.92) (90.2645, 24.323) (90.2645, 24.6522) knots 0 0 0 1 2 2 2
  spline S125 degree 2 poles (90.2645, 24.6522) (90.2645, 25.1224) (89.5424, 25.6866) (89.0823, 25.6866) knots 0 0 0 1 2 2 2
  line L175 (88.3837, 22.2911) -> (88.3837, 21.8344)
  line L176 (88.3837, 21.8344) -> (87.9169, 21.9452)
  line L177 (87.9169, 21.9452) -> (87.9169, 23.2819)
  line L178 (87.9169, 23.2819) -> (88.3837, 23.1744)
  line L179 (88.3837, 23.1744) -> (88.3837, 22.8117)
  line L180 (88.3837, 22.8117) -> (90.2175, 22.3986)
  line L181 (90.2175, 22.3986) -> (90.2175, 22.8285)
  line L182 (90.2175, 22.8285) -> (90.6843, 22.7143)
  line L183 (90.6843, 22.7143) -> (90.6843, 21.8176)
  line L184 (90.6843, 21.8176) -> (89.9018, 21.9956)
  spline S126 degree 2 poles (89.9018, 21.9956) (90.335, 21.7336) (90.728, 21.1358) (90.728, 20.7328) knots 0 0 0 1 2 2 2
  line L185 (90.728, 20.7328) -> (90.728, 20.6085)
  line L186 (90.728, 20.6085) -> (90.2175, 20.7294)
  spline S127 degree 2 poles (90.2175, 20.7294) (90.2275, 20.8067) (90.2275, 20.8604) knots 0 0 0 1 1 1
  spline S128 degree 2 poles (90.2275, 20.8604) (90.2275, 21.2265) (89.8917, 21.7605) (89.3207, 22.0795) (88.8808, 22.1803) knots 0 0 0 1 2 3 3 3
  line L187 (88.8808, 22.1803) -> (88.3837, 22.2911)
  line L188 (88.3837, 20.4507) -> (90.2175, 20.0376)
  line L189 (90.2175, 20.0376) -> (90.2175, 20.4204)
  line L190 (90.2175, 20.4204) -> (90.6843, 20.313)
  line L191 (90.6843, 20.313) -> (90.6843, 19.4162)
  line L192 (90.6843, 19.4162) -> (88.3837, 19.9335)
  line L193 (88.3837, 19.9335) -> (88.3837, 19.5304)
  line L194 (88.3837, 19.5304) -> (87.9169, 19.6413)
  line L195 (87.9169, 19.6413) -> (87.9169, 20.8638)
  line L196 (87.9169, 20.8638) -> (88.3837, 20.7563)
  line L197 (88.3837, 20.7563) -> (88.3837, 20.4507)
  spline S129 degree 2 poles (91.6381, 19.7722) (91.7725, 19.7722) (91.9639, 19.5842) (91.9639, 19.4498) knots 0 0 0 1 2 2 2
  spline S130 degree 2 poles (91.9639, 19.4498) (91.9639, 19.3155) (91.7691, 19.1308) (91.6381, 19.1308) knots 0 0 0 1 2 2 2
  spline S131 degree 2 poles (91.6381, 19.1308) (91.5038, 19.1308) (91.3124, 19.3155) (91.3124, 19.4498) knots 0 0 0 1 2 2 2
  spline S132 degree 2 poles (91.3124, 19.4498) (91.3124, 19.5808) (91.5038, 19.7722) (91.6381, 19.7722) knots 0 0 0 1 2 2 2
  line L198 (89.173, 16.2156) -> (89.173, 18.3885)
  spline S133 degree 2 poles (89.173, 18.3885) (89.089, 18.4087) (89.0151, 18.4087) knots 0 0 0 1 1 1
  spline S134 degree 2 poles (89.0151, 18.4087) (88.6726, 18.4087) (88.2897, 18.0157) (88.2897, 17.7168) knots 0 0 0 1 2 2 2
  spline S135 degree 2 poles (88.2897, 17.7168) (88.2897, 17.3037) (88.6826, 17.0149) knots 0 0 0 1 1 1
  line L199 (88.6826, 17.0149) -> (88.4509, 16.4742)
  spline S136 degree 2 poles (88.4509, 16.4742) (88.1822, 16.6387) (87.8363, 17.3239) (87.8363, 17.7135) knots 0 0 0 1 2 2 2
  spline S137 degree 2 poles (87.8363, 17.7135) (87.8363, 18.3113) (88.5281, 18.9729) (89.0689, 18.9729) knots 0 0 0 1 2 2 2
  spline S138 degree 2 poles (89.0689, 18.9729) (89.5021, 18.9729) (90.2712, 18.5363) (90.7616, 17.8041) (90.7616, 17.3675) knots 0 0 0 1 2 3 3 3
  spline S139 degree 2 poles (90.7616, 17.3675) (90.7616, 16.8403) (90.0731, 16.1753) (89.5155, 16.1753) knots 0 0 0 1 2 2 2
  spline S140 degree 2 poles (89.5155, 16.1753) (89.3375, 16.1753) (89.173, 16.2156) knots 0 0 0 1 1 1
  spline S141 degree 2 poles (89.5626, 16.7059) (89.6499, 16.6958) (89.707, 16.6958) knots 0 0 0 1 1 1
  spline S142 degree 2 poles (89.707, 16.6958) (89.9354, 16.6958) (90.3082, 17.0586) (90.3082, 17.3608) knots 0 0 0 1 2 2 2
  spline S143 degree 2 poles (90.3082, 17.3608) (90.3082, 17.6664) (89.9051, 18.1602) (89.5626, 18.2844) knots 0 0 0 1 2 2 2
  line L200 (89.5626, 18.2844) -> (89.5626, 16.7059)
  line L201 (88.6893, 15.9099) -> (88.6893, 15.4397)
  spline S144 degree 2 poles (88.6893, 15.4397) (88.4946, 15.4397) (88.283, 15.0972) (88.283, 14.8218) knots 0 0 0 1 2 2 2
  spline S145 degree 2 poles (88.283, 14.8218) (88.283, 14.5665) (88.4878, 14.2911) (88.639, 14.2911) knots 0 0 0 1 2 2 2
  spline S146 degree 2 poles (88.639, 14.2911) (88.7767, 14.2911) (88.9849, 14.5329) (89.1024, 14.8352) knots 0 0 0 1 2 2 2
  spline S147 degree 2 poles (89.1024, 14.8352) (89.22, 15.1408) (89.4081, 15.4565) (89.7406, 15.6614) (89.9286, 15.6614) knots 0 0 0 1 2 3 3 3
  spline S148 degree 2 poles (89.9286, 15.6614) (90.2477, 15.6614) (90.728, 15.1308) (90.728, 14.6639) knots 0 0 0 1 2 2 2
  spline S149 degree 2 poles (90.728, 14.6639) (90.728, 14.2307) (90.4862, 13.9486) knots 0 0 0 1 1 1
  line L202 (90.4862, 13.9486) -> (90.6843, 13.8915)
  line L203 (90.6843, 13.8915) -> (90.6843, 13.4314)
  line L204 (90.6843, 13.4314) -> (89.9152, 13.6127)
  line L205 (89.9152, 13.6127) -> (89.9152, 14.0762)
  spline S150 degree 2 poles (89.9152, 14.0762) (90.1268, 14.0829) (90.3048, 14.4523) (90.3048, 14.674) knots 0 0 0 1 2 2 2
  spline S151 degree 2 poles (90.3048, 14.674) (90.3048, 14.9024) (90.1234, 15.161) (89.9857, 15.161) knots 0 0 0 1 2 2 2
  spline S152 degree 2 poles (89.9857, 15.161) (89.8715, 15.161) (89.7271, 15.0065) (89.6432, 14.7882) knots 0 0 0 1 2 2 2
  spline S153 degree 2 poles (89.6432, 14.7882) (89.4081, 14.1702) (88.9782, 13.7773) (88.6759, 13.7773) knots 0 0 0 1 2 2 2
  spline S154 degree 2 poles (88.6759, 13.7773) (88.3132, 13.7773) (87.8699, 14.3348) (87.8699, 14.8722) knots 0 0 0 1 2 2 2
  spline S155 degree 2 poles (87.8699, 14.8722) (87.8699, 15.3759) (88.0982, 15.5842) knots 0 0 0 1 1 1
  line L206 (88.0982, 15.5842) -> (87.9169, 15.6245)
  line L207 (87.9169, 15.6245) -> (87.9169, 16.0947)
  line L208 (87.9169, 16.0947) -> (88.6893, 15.9099)
  point P0 (0, 0)
  dimension "d88" = 41.65
  dimension "d89" = 42
  dimension "d90" = 21
  constraints: 4 end point, 1 perpendicular, 1 vertical, 2 other
  measures "d88" distance of L4.end L5.end
  measures "d89" distance of L1.end L2.end
  measures "d90" distance between parallel lines of L6 L3
emboss "Inside Text" sketch "Sketch11" operation cut depth 1 direction (0, 0, -1) contours L77 L78 L67 L68 L69 L6 | L6 L69 L70 S25 S26 S27 S28 S29 S30 L72 L73 L74 L75 L76 L77 | S27 L71 S28 L6 | L7 L8 L9 L10 L11 L12 L13 L14 L15 L16 L17 L18 L19 L20 L21 L22 L23 L24 | S0 S1 S2 S3 | L25 L26 L27 L28 L29 L30 L31 L32 L33 L34 S8 L35 L36 S9 S10 L37 | L38 L39 L40 L41 S11 S12 S13 S14 L42 S15 S16 S17 L43 S18 S19 S20 L44 | L47 L48 L49 L50 L51 L52 L53 L54 L55 L56 | L57 L58 L59 L60 L61 L62 L63 L64 L65 L66 | L79 L80 L81 L82 S31 S32 S33 L83 L84 L85 L86 L87 L88 L89 L90 L91 L92 L93 S34 S35 S36 L94 | L95 S37 S38 S39 L96 S40 S41 S42 S43 S44 | L98 L99 L100 L101 L102 S48 S49 S50 S51 L103 L104 L105 L106 | L107 S56 S57 S58 L108 S59 S60 S61 S62 S63 | L110 S67 S68 S69 S70 S71 S72 L111 L112 L113 L114 S73 S74 S75 S76 S77 S78 L115 L116 L117 | L118 L119 L120 L121 S79 S80 S81 L122 S82 S83 S84 L123 L124 L125 L126 L127 L128 L129 | L130 L131 S85 S86 S87 S88 S89 L132 L133 L134 L135 L136 S90 S91 S92 L137 L138 L139 L140 L141 S93 S94 S95 L142 L143 L144 L145 L146 L147 L148 L149 L150 | L151 S96 S97 S98 L152 S99 S100 S101 S102 S103 | L154 L155 S107 S108 S109 S110 S111 L156 L157 L158 L159 L160 S112 S113 S114 L161 L162 L163 L164 L165 S115 S116 S117 L166 L167 L168 L169 L170 L171 L172 L173 L174 | S118 S119 S120 S121 | L175 L176 L177 L178 L179 L180 L181 L182 L183 L184 S126 L185 L186 S127 S128 L187 | L188 L189 L190 L191 L192 L193 L194 L195 L196 L197 | S129 S130 S131 S132 | L198 S133 S134 S135 L199 S136 S137 S138 S139 S140 | L201 S144 S145 S146 S147 S148 S149 L202 L203 L204 L205 S150 S151 S152 S153 S154 S155 L206 L207 L208
sketch "Sketch12" plane through (0, 0, 31) normal (0, 0, 1) x (1, 0, 0)
  circle A0 centre (108.3864, -12.2044) radius 1.5
  line L0 (-8.6136, -15.2044) -> (107.3864, -15.2044) projected
  line L1 (111.3864, -11.2044) -> (111.3864, 64.0956) projected
  line L2 (107.3864, -15.2044) -> (-8.6136, -15.2044) projected
  line L3 (49.3864, -15.2044) -> (49.3864, 77.1219)
  line L4 (-8.6136, -11.2044) -> (-12.6136, -11.2044) projected
  line L5 (-12.6136, -11.2044) -> (-12.6136, 26.4456)
  line L6 (-12.6136, -11.2044) -> (-12.6136, 64.0956) projected
  line L7 (-12.6136, 26.4456) -> (133.0429, 26.4456)
  circle A1 centre (-9.6136, -12.2044) radius 1.5
  line L8 (111.3864, 26.4456) -> (-34.2702, 26.4456)
  circle A2 centre (108.3864, 65.0956) radius 1.5
  line L9 (-8.6136, 64.0956) -> (-12.6136, 64.0956)
  circle A3 centre (-9.6136, 65.0956) radius 1.5
  point P0 (0, 0)
  dimension "d91" = 3
  dimension "d92" = 3
  dimension "d93" = 3
  dimension "d94" = 37.65
  constraints: 10 end point, 6 symmetric about line, 4 centre point, 2 midpoint, 2 perpendicular, 3 other
  measures "d91" diameter of A0
  measures "d92" distance from line of L0 A0.centre
  measures "d93" distance from line of L1 A0.centre
  measures "d94" distance of L4.end L5.end
extrude "3mm Screw Holes" cut sketch "Sketch12" against normal blind 10
body "Solid1"
